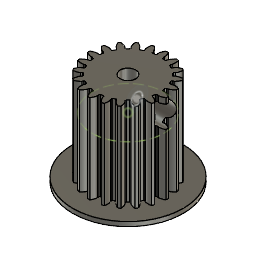
motor gear(pinion) (Autodesk Fusion 360 design; units mm, degrees)
part number: 2025-11-26-00-49-04-497
description: Spur Gear; Module: 1.617; Num Teeth: 20; Pressure Angle: 20.0; Backlash: 0.00 mm
part number: 2025-11-26-00-52-36-103
Autodesk Fusion 360 part; units mm, degrees
(part 1 of 7)
sketch "Sketch1" plane through (0, 0, 0) normal (0, 0, 1) x (1, 0, 0) in component "Spur Gear (20 teeth)"
  circle A0 centre (0, 0) radius 14.1788
  circle A1 centre (0, 0) radius 3.5
extrude "Extrude1" add sketch "Sketch1" along normal blind 15 in component "Spur Gear (20 teeth)"
sketch "Sketch2" plane through (0, 0, 0) normal (0, 0, 1) x (1, 0, 0) in component "Spur Gear (20 teeth)"
  spline S0 degree 5 poles (15.1285, -1.4178) (15.1361, -1.4185) (15.1513, -1.4197) (15.174, -1.4209) (15.2044, -1.4214) (15.2424, -1.4204) (15.2805, -1.4184) (15.3186, -1.4156) (15.3568, -1.4124) (15.395, -1.4089) (15.4332, -1.4052) (15.4714, -1.4011) (15.5096, -1.3966) (15.5478, -1.3915) (15.5861, -1.3859) (15.6243, -1.3797) (15.6625, -1.3731) (15.7008, -1.3662) (15.7391, -1.3589) (15.7773, -1.3513) (15.8155, -1.3434) (15.8538, -1.3352) (15.892, -1.3266) (15.9303, -1.3177) (15.9685, -1.3085) (16.0067, -1.2989) (16.0449, -1.2891) (16.0831, -1.2789) (16.1213, -1.2684) (16.1595, -1.2577) (16.1976, -1.2467) (16.2358, -1.2354) (16.2739, -1.2238) (16.312, -1.2119) (16.3501, -1.1998) (16.3882, -1.1874) (16.4263, -1.1747) (16.4643, -1.1618) (16.5023, -1.1486) (16.5403, -1.1351) (16.5783, -1.1214) (16.6163, -1.1075) (16.6542, -1.0933) (16.6921, -1.0789) (16.73, -1.0642) (16.7678, -1.0493) (16.8057, -1.0341) (16.8435, -1.0187) (16.8813, -1.0031) (16.919, -0.9872) (16.9567, -0.9711) (16.9944, -0.9548) (17.0321, -0.9382) (17.0697, -0.9215) (17.1073, -0.9045) (17.1449, -0.8872) (17.1824, -0.8698) (17.22, -0.8521) (17.2574, -0.8342) (17.2949, -0.8161) (17.3323, -0.7978) (17.3696, -0.7793) (17.407, -0.7606) (17.4443, -0.7416) (17.4815, -0.7225) (17.5187, -0.7031) (17.5559, -0.6835) (17.593, -0.6637) (17.6301, -0.6437) (17.6672, -0.6236) (17.7042, -0.6032) (17.7338, -0.5867) (17.756, -0.5742) (17.7707, -0.5659) (17.7781, -0.5617) knots 0 0 0 0 0 0 0.01428571 0.02857143 0.04285714 0.05714286 0.07142857 0.08571429 0.1 0.11428571 0.12857143 0.14285714 0.15714286 0.17142857 0.18571429 0.2 0.21428571 0.22857143 0.24285714 0.25714286 0.27142857 0.28571429 0.3 0.31428571 0.32857143 0.34285714 0.35714286 0.37142857 0.38571429 0.4 0.41428571 0.42857143 0.44285714 0.45714286 0.47142857 0.48571429 0.5 0.51428571 0.52857143 0.54285714 0.55714286 0.57142857 0.58571429 0.6 0.61428571 0.62857143 0.64285714 0.65714286 0.67142857 0.68571429 0.7 0.71428571 0.72857143 0.74285714 0.75714286 0.77142857 0.78571429 0.8 0.81428571 0.82857143 0.84285714 0.85714286 0.87142857 0.88571429 0.9 0.91428571 0.92857143 0.94285714 0.95714286 0.97142857 0.98571429 1 1 1 1 1 1
  spline S1 degree 5 poles (15.1285, 1.4178) (15.1361, 1.4185) (15.1513, 1.4197) (15.174, 1.4209) (15.2044, 1.4214) (15.2424, 1.4204) (15.2805, 1.4184) (15.3186, 1.4156) (15.3568, 1.4124) (15.395, 1.4089) (15.4332, 1.4052) (15.4714, 1.4011) (15.5096, 1.3966) (15.5478, 1.3915) (15.5861, 1.3859) (15.6243, 1.3797) (15.6625, 1.3731) (15.7008, 1.3662) (15.7391, 1.3589) (15.7773, 1.3513) (15.8155, 1.3434) (15.8538, 1.3352) (15.892, 1.3266) (15.9303, 1.3177) (15.9685, 1.3085) (16.0067, 1.2989) (16.0449, 1.2891) (16.0831, 1.2789) (16.1213, 1.2684) (16.1595, 1.2577) (16.1976, 1.2467) (16.2358, 1.2354) (16.2739, 1.2238) (16.312, 1.2119) (16.3501, 1.1998) (16.3882, 1.1874) (16.4263, 1.1747) (16.4643, 1.1618) (16.5023, 1.1486) (16.5403, 1.1351) (16.5783, 1.1214) (16.6163, 1.1075) (16.6542, 1.0933) (16.6921, 1.0789) (16.73, 1.0642) (16.7678, 1.0493) (16.8057, 1.0341) (16.8435, 1.0187) (16.8813, 1.0031) (16.919, 0.9872) (16.9567, 0.9711) (16.9944, 0.9548) (17.0321, 0.9382) (17.0697, 0.9215) (17.1073, 0.9045) (17.1449, 0.8872) (17.1824, 0.8698) (17.22, 0.8521) (17.2574, 0.8342) (17.2949, 0.8161) (17.3323, 0.7978) (17.3696, 0.7793) (17.407, 0.7606) (17.4443, 0.7416) (17.4815, 0.7225) (17.5187, 0.7031) (17.5559, 0.6835) (17.593, 0.6637) (17.6301, 0.6437) (17.6672, 0.6236) (17.7042, 0.6032) (17.7338, 0.5867) (17.756, 0.5742) (17.7707, 0.5659) (17.7781, 0.5617) knots 0 0 0 0 0 0 0.01428571 0.02857143 0.04285714 0.05714286 0.07142857 0.08571429 0.1 0.11428571 0.12857143 0.14285714 0.15714286 0.17142857 0.18571429 0.2 0.21428571 0.22857143 0.24285714 0.25714286 0.27142857 0.28571429 0.3 0.31428571 0.32857143 0.34285714 0.35714286 0.37142857 0.38571429 0.4 0.41428571 0.42857143 0.44285714 0.45714286 0.47142857 0.48571429 0.5 0.51428571 0.52857143 0.54285714 0.55714286 0.57142857 0.58571429 0.6 0.61428571 0.62857143 0.64285714 0.65714286 0.67142857 0.68571429 0.7 0.71428571 0.72857143 0.74285714 0.75714286 0.77142857 0.78571429 0.8 0.81428571 0.82857143 0.84285714 0.85714286 0.87142857 0.88571429 0.9 0.91428571 0.92857143 0.94285714 0.95714286 0.97142857 0.98571429 1 1 1 1 1 1
  arc A0 (17.7781, -0.5617) -> (17.7781, 0.5617) centre (0, 0) ccw
  line L0 (14.107, -1.323) -> (15.1285, -1.4178)
  line L1 (14.107, 1.323) -> (15.1285, 1.4178)
  line L2 (14.107, -1.323) -> (14.107, 1.323)
  point P0 (15.3147, -1.4158)
  point P1 (15.5023, -1.3974)
  point P2 (15.6908, -1.3679)
  point P3 (15.8799, -1.3293)
  point P4 (16.0695, -1.2825)
  point P5 (16.2594, -1.2281)
  point P6 (16.4496, -1.1667)
  point P7 (16.6398, -1.0986)
  point P8 (16.8301, -1.0241)
  point P9 (17.0203, -0.9434)
  point P10 (17.2102, -0.8567)
  point P11 (17.3999, -0.7641)
  point P12 (17.5893, -0.6657)
  point P13 (15.3147, 1.4158)
  point P14 (15.5023, 1.3974)
  point P15 (15.6908, 1.3679)
  point P16 (15.8799, 1.3293)
  point P17 (16.0695, 1.2825)
  point P18 (16.2594, 1.2281)
  point P19 (16.4496, 1.1667)
  point P20 (16.6398, 1.0986)
  point P21 (16.8301, 1.0241)
  point P22 (17.0203, 0.9434)
  point P23 (17.2102, 0.8567)
  point P24 (17.3999, 0.7641)
  point P25 (17.5893, 0.6657)
extrude "Extrude2" add sketch "Sketch2" along normal blind 15 in component "Spur Gear (20 teeth)"
fillet "Fillet1" radius 0.4 2 edges at (14.1169, -1.3239, 7.5) (14.1169, 1.3239, 7.5) in component "Spur Gear (20 teeth)"
pattern_circular "C-Pattern1" count 20 over 360 about axis through (0, 0, 0) along (0, 0, 1) of "Extrude2", "Fillet1" in component "Spur Gear (20 teeth)"
sketch "Sketch3" plane through (0, 0, 0) normal (0, 0, 1) x (1, 0, 0) in component "Spur Gear (20 teeth)"
  circle A0 centre (0, 0) radius 16.17 construction
sketch "Sketch1 (2)" plane through (0, 0, 0) normal (1, 0, 0) x (0, 1, 0)
  circle A0 through (5, 7.5, 4) (-2.5, 11.8301, 4) (-2.5, 3.1699, 4)
  dimension "d9" = 10
sketch "Sketch2 (2)" plane through (4, 0, 0) normal (1, 0, 0) x (0, 1, 0)
extrude "Extrude7" cut sketch "Sketch1 (2)" along normal blind 16 contours A0 in plane through (4, 0, 0) normal (1, 0, 0) in component "Spur Gear (20 teeth)"
sketch "Sketch4" plane through (4, 0, 0) normal (1, 0, 0) x (0, 1, 0)
  circle A0 centre (0, 7.5) radius 5
  circle A1 centre (0, 7.5) radius 2.5
  dimension "d21" = 5
  constraint concentric A0 A1
  measures "d21" diameter of A1
extrude "Extrude8" cut sketch "Sketch4" against normal blind 16 contours A1 in component "Spur Gear (20 teeth)"
extrude "Extrude10" add 1 faces at (10.5636, 0, 0) along direction (0, 0, -1) blind 10 in component "Spur Gear (20 teeth)"
sketch "Sketch7" plane through (0, 0, -10) normal (0, 0, -1) x (1, 0, 0)
  circle A0 centre (0, 0) radius 3.5
  arc A1 (12.5379, 7.4278) -> (12.3925, 6.8895) centre (12.7421, 7.0839) ccw
  line L0 (12.5379, 7.4278) -> (13.0726, 7.7453)
  spline S0 degree 5 poles (13.0726, 7.7453) (13.0791, 7.7492) (13.0921, 7.7571) (13.1112, 7.7695) (13.1361, 7.787) (13.1663, 7.8101) (13.1959, 7.8342) (13.2251, 7.8589) (13.2541, 7.8839) (13.2829, 7.9091) (13.3116, 7.9346) (13.3402, 7.9603) (13.3684, 7.9864) (13.3963, 8.013) (13.424, 8.0401) (13.4513, 8.0675) (13.4784, 8.0953) (13.5052, 8.1235) (13.5319, 8.1518) (13.5584, 8.1805) (13.5847, 8.2093) (13.6108, 8.2384) (13.6367, 8.2678) (13.6624, 8.2975) (13.6879, 8.3274) (13.7132, 8.3576) (13.7383, 8.3881) (13.7632, 8.4188) (13.788, 8.4497) (13.8125, 8.4808) (13.8369, 8.5122) (13.8611, 8.5437) (13.8852, 8.5755) (13.909, 8.6075) (13.9327, 8.6397) (13.9562, 8.6721) (13.9796, 8.7048) (14.0028, 8.7376) (14.0258, 8.7706) (14.0486, 8.8038) (14.0713, 8.8372) (14.0938, 8.8708) (14.1162, 8.9046) (14.1383, 8.9386) (14.1604, 8.9727) (14.1822, 9.007) (14.2039, 9.0415) (14.2254, 9.0762) (14.2468, 9.1111) (14.268, 9.1461) (14.2891, 9.1813) (14.31, 9.2166) (14.3307, 9.2522) (14.3513, 9.2879) (14.3718, 9.3237) (14.392, 9.3597) (14.4121, 9.3959) (14.4321, 9.4323) (14.4519, 9.4687) (14.4716, 9.5054) (14.491, 9.5422) (14.5104, 9.5791) (14.5296, 9.6162) (14.5486, 9.6535) (14.5675, 9.6909) (14.5862, 9.7284) (14.6048, 9.7661) (14.6232, 9.804) (14.6415, 9.8419) (14.6596, 9.8801) (14.6775, 9.9183) (14.6918, 9.949) (14.7024, 9.9721) (14.7095, 9.9876) (14.713, 9.9953) knots 0 0 0 0 0 0 0.01428571 0.02857143 0.04285714 0.05714286 0.07142857 0.08571429 0.1 0.11428571 0.12857143 0.14285714 0.15714286 0.17142857 0.18571429 0.2 0.21428571 0.22857143 0.24285714 0.25714286 0.27142857 0.28571429 0.3 0.31428571 0.32857143 0.34285714 0.35714286 0.37142857 0.38571429 0.4 0.41428571 0.42857143 0.44285714 0.45714286 0.47142857 0.48571429 0.5 0.51428571 0.52857143 0.54285714 0.55714286 0.57142857 0.58571429 0.6 0.61428571 0.62857143 0.64285714 0.65714286 0.67142857 0.68571429 0.7 0.71428571 0.72857143 0.74285714 0.75714286 0.77142857 0.78571429 0.8 0.81428571 0.82857143 0.84285714 0.85714286 0.87142857 0.88571429 0.9 0.91428571 0.92857143 0.94285714 0.95714286 0.97142857 0.98571429 1 1 1 1 1 1
  arc A2 (14.713, 9.9953) -> (14.0526, 10.9042) centre (0, 0) ccw
  spline S1 degree 5 poles (14.0526, 10.9042) (14.0442, 10.9032) (14.0274, 10.9013) (14.0021, 10.8983) (13.9685, 10.8942) (13.9266, 10.889) (13.8847, 10.8835) (13.8429, 10.8779) (13.8013, 10.8721) (13.7597, 10.8661) (13.7182, 10.8598) (13.6768, 10.8535) (13.6355, 10.8469) (13.5943, 10.8401) (13.5531, 10.8331) (13.5121, 10.8259) (13.4712, 10.8186) (13.4304, 10.811) (13.3896, 10.8033) (13.349, 10.7953) (13.3085, 10.7872) (13.2681, 10.7788) (13.2278, 10.7703) (13.1876, 10.7615) (13.1475, 10.7526) (13.1075, 10.7434) (13.0676, 10.7341) (13.0279, 10.7245) (12.9883, 10.7147) (12.9487, 10.7048) (12.9093, 10.6946) (12.8701, 10.6842) (12.8309, 10.6736) (12.7919, 10.6628) (12.753, 10.6517) (12.7142, 10.6405) (12.6755, 10.629) (12.637, 10.6174) (12.5987, 10.6055) (12.5604, 10.5933) (12.5223, 10.581) (12.4844, 10.5684) (12.4466, 10.5556) (12.4089, 10.5426) (12.3714, 10.5293) (12.334, 10.5158) (12.2968, 10.502) (12.2598, 10.4881) (12.2229, 10.4738) (12.1862, 10.4594) (12.1497, 10.4446) (12.1133, 10.4296) (12.0772, 10.4144) (12.0412, 10.3988) (12.0054, 10.383) (11.9698, 10.3669) (11.9344, 10.3505) (11.8992, 10.3339) (11.8642, 10.3171) (11.8294, 10.2999) (11.7948, 10.2824) (11.7605, 10.2645) (11.7266, 10.2462) (11.693, 10.2274) (11.6597, 10.2082) (11.6266, 10.1888) (11.5937, 10.1691) (11.561, 10.1493) (11.5285, 10.1291) (11.4965, 10.1084) (11.4651, 10.0869) (11.4408, 10.0686) (11.4231, 10.0543) (11.4116, 10.0444) (11.4059, 10.0394) knots -1 -1 -1 -1 -1 -1 -0.98571429 -0.97142857 -0.95714286 -0.94285714 -0.92857143 -0.91428571 -0.9 -0.88571429 -0.87142857 -0.85714286 -0.84285714 -0.82857143 -0.81428571 -0.8 -0.78571429 -0.77142857 -0.75714286 -0.74285714 -0.72857143 -0.71428571 -0.7 -0.68571429 -0.67142857 -0.65714286 -0.64285714 -0.62857143 -0.61428571 -0.6 -0.58571429 -0.57142857 -0.55714286 -0.54285714 -0.52857143 -0.51428571 -0.5 -0.48571429 -0.47142857 -0.45714286 -0.44285714 -0.42857143 -0.41428571 -0.4 -0.38571429 -0.37142857 -0.35714286 -0.34285714 -0.32857143 -0.31428571 -0.3 -0.28571429 -0.27142857 -0.25714286 -0.24285714 -0.22857143 -0.21428571 -0.2 -0.18571429 -0.17142857 -0.15714286 -0.14285714 -0.12857143 -0.11428571 -0.1 -0.08571429 -0.07142857 -0.05714286 -0.04285714 -0.02857143 -0.01428571 0 0 0 0 0 0
  line L1 (11.4059, 10.0394) -> (10.9387, 9.6289)
  arc A3 (10.3818, 9.657) -> (10.9387, 9.6289) centre (10.6747, 9.9294) ccw
  arc A4 (10.3818, 9.657) -> (9.657, 10.3818) centre (0, 0) ccw
  arc A5 (9.6289, 10.9387) -> (9.657, 10.3818) centre (9.9294, 10.6747) ccw
  line L2 (9.6289, 10.9387) -> (10.0394, 11.4059)
  spline S2 degree 5 poles (10.0394, 11.4059) (10.0444, 11.4116) (10.0543, 11.4231) (10.0686, 11.4408) (10.0869, 11.4651) (10.1084, 11.4965) (10.1291, 11.5285) (10.1493, 11.561) (10.1691, 11.5937) (10.1888, 11.6266) (10.2082, 11.6597) (10.2274, 11.693) (10.2462, 11.7266) (10.2645, 11.7605) (10.2824, 11.7948) (10.2999, 11.8294) (10.3171, 11.8642) (10.3339, 11.8992) (10.3505, 11.9344) (10.3669, 11.9698) (10.383, 12.0054) (10.3988, 12.0412) (10.4144, 12.0772) (10.4296, 12.1133) (10.4446, 12.1497) (10.4594, 12.1862) (10.4738, 12.2229) (10.4881, 12.2598) (10.502, 12.2968) (10.5158, 12.334) (10.5293, 12.3714) (10.5426, 12.4089) (10.5556, 12.4466) (10.5684, 12.4844) (10.581, 12.5223) (10.5933, 12.5604) (10.6055, 12.5987) (10.6174, 12.637) (10.629, 12.6755) (10.6405, 12.7142) (10.6517, 12.753) (10.6628, 12.7919) (10.6736, 12.8309) (10.6842, 12.8701) (10.6946, 12.9093) (10.7048, 12.9487) (10.7147, 12.9883) (10.7245, 13.0279) (10.7341, 13.0676) (10.7434, 13.1075) (10.7526, 13.1475) (10.7615, 13.1876) (10.7703, 13.2278) (10.7788, 13.2681) (10.7872, 13.3085) (10.7953, 13.349) (10.8033, 13.3896) (10.811, 13.4304) (10.8186, 13.4712) (10.8259, 13.5121) (10.8331, 13.5531) (10.8401, 13.5943) (10.8469, 13.6355) (10.8535, 13.6768) (10.8598, 13.7182) (10.8661, 13.7597) (10.8721, 13.8013) (10.8779, 13.8429) (10.8835, 13.8847) (10.889, 13.9266) (10.8942, 13.9685) (10.8983, 14.0021) (10.9013, 14.0274) (10.9032, 14.0442) (10.9042, 14.0526) knots 0 0 0 0 0 0 0.01428571 0.02857143 0.04285714 0.05714286 0.07142857 0.08571429 0.1 0.11428571 0.12857143 0.14285714 0.15714286 0.17142857 0.18571429 0.2 0.21428571 0.22857143 0.24285714 0.25714286 0.27142857 0.28571429 0.3 0.31428571 0.32857143 0.34285714 0.35714286 0.37142857 0.38571429 0.4 0.41428571 0.42857143 0.44285714 0.45714286 0.47142857 0.48571429 0.5 0.51428571 0.52857143 0.54285714 0.55714286 0.57142857 0.58571429 0.6 0.61428571 0.62857143 0.64285714 0.65714286 0.67142857 0.68571429 0.7 0.71428571 0.72857143 0.74285714 0.75714286 0.77142857 0.78571429 0.8 0.81428571 0.82857143 0.84285714 0.85714286 0.87142857 0.88571429 0.9 0.91428571 0.92857143 0.94285714 0.95714286 0.97142857 0.98571429 1 1 1 1 1 1
  arc A6 (10.9042, 14.0526) -> (9.9953, 14.713) centre (0, 0) ccw
  spline S3 degree 5 poles (9.9953, 14.713) (9.9876, 14.7095) (9.9721, 14.7024) (9.949, 14.6918) (9.9183, 14.6775) (9.8801, 14.6596) (9.8419, 14.6415) (9.804, 14.6232) (9.7661, 14.6048) (9.7284, 14.5862) (9.6909, 14.5675) (9.6535, 14.5486) (9.6162, 14.5296) (9.5791, 14.5104) (9.5422, 14.491) (9.5054, 14.4716) (9.4687, 14.4519) (9.4323, 14.4321) (9.3959, 14.4121) (9.3597, 14.392) (9.3237, 14.3718) (9.2879, 14.3513) (9.2522, 14.3307) (9.2166, 14.31) (9.1813, 14.2891) (9.1461, 14.268) (9.1111, 14.2468) (9.0762, 14.2254) (9.0415, 14.2039) (9.007, 14.1822) (8.9727, 14.1604) (8.9386, 14.1383) (8.9046, 14.1162) (8.8708, 14.0938) (8.8372, 14.0713) (8.8038, 14.0486) (8.7706, 14.0258) (8.7376, 14.0028) (8.7048, 13.9796) (8.6721, 13.9562) (8.6397, 13.9327) (8.6075, 13.909) (8.5755, 13.8852) (8.5437, 13.8611) (8.5122, 13.8369) (8.4808, 13.8125) (8.4497, 13.788) (8.4188, 13.7632) (8.3881, 13.7383) (8.3576, 13.7132) (8.3274, 13.6879) (8.2975, 13.6624) (8.2678, 13.6367) (8.2384, 13.6108) (8.2093, 13.5847) (8.1805, 13.5584) (8.1518, 13.5319) (8.1235, 13.5052) (8.0953, 13.4784) (8.0675, 13.4513) (8.0401, 13.424) (8.013, 13.3963) (7.9864, 13.3684) (7.9603, 13.3402) (7.9346, 13.3116) (7.9091, 13.2829) (7.8839, 13.2541) (7.8589, 13.2251) (7.8342, 13.1959) (7.8101, 13.1663) (7.787, 13.1361) (7.7695, 13.1112) (7.7571, 13.0921) (7.7492, 13.0791) (7.7453, 13.0726) knots -1 -1 -1 -1 -1 -1 -0.98571429 -0.97142857 -0.95714286 -0.94285714 -0.92857143 -0.91428571 -0.9 -0.88571429 -0.87142857 -0.85714286 -0.84285714 -0.82857143 -0.81428571 -0.8 -0.78571429 -0.77142857 -0.75714286 -0.74285714 -0.72857143 -0.71428571 -0.7 -0.68571429 -0.67142857 -0.65714286 -0.64285714 -0.62857143 -0.61428571 -0.6 -0.58571429 -0.57142857 -0.55714286 -0.54285714 -0.52857143 -0.51428571 -0.5 -0.48571429 -0.47142857 -0.45714286 -0.44285714 -0.42857143 -0.41428571 -0.4 -0.38571429 -0.37142857 -0.35714286 -0.34285714 -0.32857143 -0.31428571 -0.3 -0.28571429 -0.27142857 -0.25714286 -0.24285714 -0.22857143 -0.21428571 -0.2 -0.18571429 -0.17142857 -0.15714286 -0.14285714 -0.12857143 -0.11428571 -0.1 -0.08571429 -0.07142857 -0.05714286 -0.04285714 -0.02857143 -0.01428571 0 0 0 0 0 0
  line L3 (7.7453, 13.0726) -> (7.4278, 12.5379)
  arc A7 (6.8895, 12.3925) -> (7.4278, 12.5379) centre (7.0839, 12.7421) ccw
  arc A8 (6.8895, 12.3925) -> (5.9762, 12.8578) centre (0, 0) ccw
  arc A9 (5.7774, 13.3788) -> (5.9762, 12.8578) centre (6.1448, 13.2206) ccw
  line L4 (5.7774, 13.3788) -> (6.0234, 13.95)
  spline S4 degree 5 poles (6.0234, 13.95) (6.0264, 13.957) (6.0322, 13.971) (6.0404, 13.9923) (6.0502, 14.021) (6.0611, 14.0575) (6.0709, 14.0943) (6.08, 14.1315) (6.0888, 14.1687) (6.0973, 14.2061) (6.1055, 14.2436) (6.1135, 14.2812) (6.121, 14.3189) (6.1279, 14.3569) (6.1344, 14.395) (6.1404, 14.4332) (6.1459, 14.4717) (6.1511, 14.5102) (6.156, 14.5488) (6.1606, 14.5875) (6.1649, 14.6264) (6.1689, 14.6653) (6.1726, 14.7043) (6.176, 14.7434) (6.179, 14.7826) (6.1817, 14.8219) (6.1841, 14.8613) (6.1862, 14.9008) (6.1881, 14.9403) (6.1897, 14.9799) (6.191, 15.0196) (6.192, 15.0594) (6.1928, 15.0992) (6.1933, 15.1392) (6.1935, 15.1791) (6.1935, 15.2192) (6.1932, 15.2593) (6.1927, 15.2995) (6.1919, 15.3397) (6.1908, 15.38) (6.1895, 15.4204) (6.188, 15.4608) (6.1862, 15.5012) (6.1842, 15.5417) (6.182, 15.5823) (6.1795, 15.6229) (6.1767, 15.6636) (6.1738, 15.7043) (6.1706, 15.7451) (6.1672, 15.7859) (6.1635, 15.8267) (6.1596, 15.8676) (6.1555, 15.9086) (6.1512, 15.9495) (6.1466, 15.9906) (6.1419, 16.0316) (6.1369, 16.0727) (6.1317, 16.1138) (6.1262, 16.155) (6.1206, 16.1962) (6.1147, 16.2374) (6.1087, 16.2787) (6.1024, 16.32) (6.0959, 16.3613) (6.0892, 16.4027) (6.0823, 16.444) (6.0751, 16.4854) (6.0678, 16.5269) (6.0602, 16.5683) (6.0525, 16.6098) (6.0445, 16.6513) (6.038, 16.6846) (6.033, 16.7095) (6.0297, 16.7261) (6.028, 16.7344) knots 0 0 0 0 0 0 0.01428571 0.02857143 0.04285714 0.05714286 0.07142857 0.08571429 0.1 0.11428571 0.12857143 0.14285714 0.15714286 0.17142857 0.18571429 0.2 0.21428571 0.22857143 0.24285714 0.25714286 0.27142857 0.28571429 0.3 0.31428571 0.32857143 0.34285714 0.35714286 0.37142857 0.38571429 0.4 0.41428571 0.42857143 0.44285714 0.45714286 0.47142857 0.48571429 0.5 0.51428571 0.52857143 0.54285714 0.55714286 0.57142857 0.58571429 0.6 0.61428571 0.62857143 0.64285714 0.65714286 0.67142857 0.68571429 0.7 0.71428571 0.72857143 0.74285714 0.75714286 0.77142857 0.78571429 0.8 0.81428571 0.82857143 0.84285714 0.85714286 0.87142857 0.88571429 0.9 0.91428571 0.92857143 0.94285714 0.95714286 0.97142857 0.98571429 1 1 1 1 1 1
  arc A10 (6.028, 16.7344) -> (4.9595, 17.0816) centre (0, 0) ccw
  spline S5 degree 5 poles (4.9595, 17.0816) (4.9533, 17.0759) (4.9408, 17.0644) (4.9221, 17.0471) (4.8973, 17.0241) (4.8664, 16.9952) (4.8358, 16.9662) (4.8053, 16.9371) (4.775, 16.9079) (4.7449, 16.8786) (4.715, 16.8492) (4.6853, 16.8196) (4.6557, 16.79) (4.6263, 16.7603) (4.5972, 16.7305) (4.5682, 16.7006) (4.5394, 16.6706) (4.5108, 16.6405) (4.4825, 16.6103) (4.4543, 16.5799) (4.4263, 16.5495) (4.3985, 16.519) (4.3709, 16.4884) (4.3435, 16.4577) (4.3163, 16.4269) (4.2894, 16.396) (4.2626, 16.365) (4.2361, 16.3339) (4.2098, 16.3027) (4.1836, 16.2714) (4.1577, 16.24) (4.1321, 16.2085) (4.1066, 16.1769) (4.0814, 16.1452) (4.0564, 16.1134) (4.0317, 16.0816) (4.0071, 16.0496) (3.9828, 16.0175) (3.9588, 15.9853) (3.935, 15.953) (3.9114, 15.9206) (3.8881, 15.8882) (3.865, 15.8556) (3.8422, 15.8229) (3.8197, 15.7901) (3.7974, 15.7572) (3.7754, 15.7242) (3.7537, 15.6911) (3.7322, 15.658) (3.711, 15.6247) (3.6901, 15.5913) (3.6695, 15.5578) (3.6492, 15.5242) (3.6293, 15.4904) (3.6096, 15.4566) (3.5903, 15.4227) (3.5713, 15.3886) (3.5525, 15.3545) (3.5341, 15.3203) (3.516, 15.2859) (3.4983, 15.2515) (3.4811, 15.2168) (3.4645, 15.1821) (3.4484, 15.1471) (3.4327, 15.112) (3.4173, 15.0769) (3.4023, 15.0416) (3.3874, 15.0063) (3.373, 14.9709) (3.3592, 14.9353) (3.3466, 14.8995) (3.3376, 14.8704) (3.3318, 14.8484) (3.3282, 14.8336) (3.3266, 14.8262) knots -1 -1 -1 -1 -1 -1 -0.98571429 -0.97142857 -0.95714286 -0.94285714 -0.92857143 -0.91428571 -0.9 -0.88571429 -0.87142857 -0.85714286 -0.84285714 -0.82857143 -0.81428571 -0.8 -0.78571429 -0.77142857 -0.75714286 -0.74285714 -0.72857143 -0.71428571 -0.7 -0.68571429 -0.67142857 -0.65714286 -0.64285714 -0.62857143 -0.61428571 -0.6 -0.58571429 -0.57142857 -0.55714286 -0.54285714 -0.52857143 -0.51428571 -0.5 -0.48571429 -0.47142857 -0.45714286 -0.44285714 -0.42857143 -0.41428571 -0.4 -0.38571429 -0.37142857 -0.35714286 -0.34285714 -0.32857143 -0.31428571 -0.3 -0.28571429 -0.27142857 -0.25714286 -0.24285714 -0.22857143 -0.21428571 -0.2 -0.18571429 -0.17142857 -0.15714286 -0.14285714 -0.12857143 -0.11428571 -0.1 -0.08571429 -0.07142857 -0.05714286 -0.04285714 -0.02857143 -0.01428571 0 0 0 0 0 0
  line L5 (3.3266, 14.8262) -> (3.1899, 14.2195)
  arc A11 (2.7228, 13.9149) -> (3.1899, 14.2195) centre (2.7996, 14.3075) ccw
  arc A12 (2.7228, 13.9149) -> (1.7104, 14.0753) centre (0, 0) ccw
  arc A13 (1.3603, 14.5093) -> (1.7104, 14.0753) centre (1.7586, 14.4723) ccw
  line L6 (1.3603, 14.5093) -> (1.4178, 15.1285)
  spline S6 degree 5 poles (1.4178, 15.1285) (1.4185, 15.1361) (1.4197, 15.1513) (1.4209, 15.174) (1.4214, 15.2044) (1.4204, 15.2424) (1.4184, 15.2805) (1.4156, 15.3186) (1.4124, 15.3568) (1.4089, 15.395) (1.4052, 15.4332) (1.4011, 15.4714) (1.3966, 15.5096) (1.3915, 15.5478) (1.3859, 15.5861) (1.3797, 15.6243) (1.3731, 15.6625) (1.3662, 15.7008) (1.3589, 15.7391) (1.3513, 15.7773) (1.3434, 15.8155) (1.3352, 15.8538) (1.3266, 15.892) (1.3177, 15.9303) (1.3085, 15.9685) (1.2989, 16.0067) (1.2891, 16.0449) (1.2789, 16.0831) (1.2684, 16.1213) (1.2577, 16.1595) (1.2467, 16.1976) (1.2354, 16.2358) (1.2238, 16.2739) (1.2119, 16.312) (1.1998, 16.3501) (1.1874, 16.3882) (1.1747, 16.4263) (1.1618, 16.4643) (1.1486, 16.5023) (1.1351, 16.5403) (1.1214, 16.5783) (1.1075, 16.6163) (1.0933, 16.6542) (1.0789, 16.6921) (1.0642, 16.73) (1.0493, 16.7678) (1.0341, 16.8057) (1.0187, 16.8435) (1.0031, 16.8813) (0.9872, 16.919) (0.9711, 16.9567) (0.9548, 16.9944) (0.9382, 17.0321) (0.9215, 17.0697) (0.9045, 17.1073) (0.8872, 17.1449) (0.8698, 17.1824) (0.8521, 17.22) (0.8342, 17.2574) (0.8161, 17.2949) (0.7978, 17.3323) (0.7793, 17.3696) (0.7606, 17.407) (0.7416, 17.4443) (0.7225, 17.4815) (0.7031, 17.5187) (0.6835, 17.5559) (0.6637, 17.593) (0.6437, 17.6301) (0.6236, 17.6672) (0.6032, 17.7042) (0.5867, 17.7338) (0.5742, 17.756) (0.5659, 17.7707) (0.5617, 17.7781) knots 0 0 0 0 0 0 0.01428571 0.02857143 0.04285714 0.05714286 0.07142857 0.08571429 0.1 0.11428571 0.12857143 0.14285714 0.15714286 0.17142857 0.18571429 0.2 0.21428571 0.22857143 0.24285714 0.25714286 0.27142857 0.28571429 0.3 0.31428571 0.32857143 0.34285714 0.35714286 0.37142857 0.38571429 0.4 0.41428571 0.42857143 0.44285714 0.45714286 0.47142857 0.48571429 0.5 0.51428571 0.52857143 0.54285714 0.55714286 0.57142857 0.58571429 0.6 0.61428571 0.62857143 0.64285714 0.65714286 0.67142857 0.68571429 0.7 0.71428571 0.72857143 0.74285714 0.75714286 0.77142857 0.78571429 0.8 0.81428571 0.82857143 0.84285714 0.85714286 0.87142857 0.88571429 0.9 0.91428571 0.92857143 0.94285714 0.95714286 0.97142857 0.98571429 1 1 1 1 1 1
  arc A14 (0.5617, 17.7781) -> (-0.5617, 17.7781) centre (0, 0) ccw
  spline S7 degree 5 poles (-0.5617, 17.7781) (-0.5659, 17.7707) (-0.5742, 17.756) (-0.5867, 17.7338) (-0.6032, 17.7042) (-0.6236, 17.6672) (-0.6437, 17.6301) (-0.6637, 17.593) (-0.6835, 17.5559) (-0.7031, 17.5187) (-0.7225, 17.4815) (-0.7416, 17.4443) (-0.7606, 17.407) (-0.7793, 17.3696) (-0.7978, 17.3323) (-0.8161, 17.2949) (-0.8342, 17.2574) (-0.8521, 17.22) (-0.8698, 17.1824) (-0.8872, 17.1449) (-0.9045, 17.1073) (-0.9215, 17.0697) (-0.9382, 17.0321) (-0.9548, 16.9944) (-0.9711, 16.9567) (-0.9872, 16.919) (-1.0031, 16.8813) (-1.0187, 16.8435) (-1.0341, 16.8057) (-1.0493, 16.7678) (-1.0642, 16.73) (-1.0789, 16.6921) (-1.0933, 16.6542) (-1.1075, 16.6163) (-1.1214, 16.5783) (-1.1351, 16.5403) (-1.1486, 16.5023) (-1.1618, 16.4643) (-1.1747, 16.4263) (-1.1874, 16.3882) (-1.1998, 16.3501) (-1.2119, 16.312) (-1.2238, 16.2739) (-1.2354, 16.2358) (-1.2467, 16.1976) (-1.2577, 16.1595) (-1.2684, 16.1213) (-1.2789, 16.0831) (-1.2891, 16.0449) (-1.2989, 16.0067) (-1.3085, 15.9685) (-1.3177, 15.9303) (-1.3266, 15.892) (-1.3352, 15.8538) (-1.3434, 15.8155) (-1.3513, 15.7773) (-1.3589, 15.7391) (-1.3662, 15.7008) (-1.3731, 15.6625) (-1.3797, 15.6243) (-1.3859, 15.5861) (-1.3915, 15.5478) (-1.3966, 15.5096) (-1.4011, 15.4714) (-1.4052, 15.4332) (-1.4089, 15.395) (-1.4124, 15.3568) (-1.4156, 15.3186) (-1.4184, 15.2805) (-1.4204, 15.2424) (-1.4214, 15.2044) (-1.4209, 15.174) (-1.4197, 15.1513) (-1.4185, 15.1361) (-1.4178, 15.1285) knots -1 -1 -1 -1 -1 -1 -0.98571429 -0.97142857 -0.95714286 -0.94285714 -0.92857143 -0.91428571 -0.9 -0.88571429 -0.87142857 -0.85714286 -0.84285714 -0.82857143 -0.81428571 -0.8 -0.78571429 -0.77142857 -0.75714286 -0.74285714 -0.72857143 -0.71428571 -0.7 -0.68571429 -0.67142857 -0.65714286 -0.64285714 -0.62857143 -0.61428571 -0.6 -0.58571429 -0.57142857 -0.55714286 -0.54285714 -0.52857143 -0.51428571 -0.5 -0.48571429 -0.47142857 -0.45714286 -0.44285714 -0.42857143 -0.41428571 -0.4 -0.38571429 -0.37142857 -0.35714286 -0.34285714 -0.32857143 -0.31428571 -0.3 -0.28571429 -0.27142857 -0.25714286 -0.24285714 -0.22857143 -0.21428571 -0.2 -0.18571429 -0.17142857 -0.15714286 -0.14285714 -0.12857143 -0.11428571 -0.1 -0.08571429 -0.07142857 -0.05714286 -0.04285714 -0.02857143 -0.01428571 0 0 0 0 0 0
  line L7 (-1.4178, 15.1285) -> (-1.3603, 14.5093)
  arc A15 (-1.7104, 14.0753) -> (-1.3603, 14.5093) centre (-1.7586, 14.4723) ccw
  arc A16 (-1.7104, 14.0753) -> (-2.7228, 13.9149) centre (0, 0) ccw
  arc A17 (-3.1899, 14.2195) -> (-2.7228, 13.9149) centre (-2.7996, 14.3075) ccw
  line L8 (-3.1899, 14.2195) -> (-3.3266, 14.8262)
  spline S8 degree 5 poles (-3.3266, 14.8262) (-3.3282, 14.8336) (-3.3318, 14.8484) (-3.3376, 14.8704) (-3.3466, 14.8995) (-3.3592, 14.9353) (-3.373, 14.9709) (-3.3874, 15.0063) (-3.4023, 15.0416) (-3.4173, 15.0769) (-3.4327, 15.112) (-3.4484, 15.1471) (-3.4645, 15.1821) (-3.4811, 15.2168) (-3.4983, 15.2515) (-3.516, 15.2859) (-3.5341, 15.3203) (-3.5525, 15.3545) (-3.5713, 15.3886) (-3.5903, 15.4227) (-3.6096, 15.4566) (-3.6293, 15.4904) (-3.6492, 15.5242) (-3.6695, 15.5578) (-3.6901, 15.5913) (-3.711, 15.6247) (-3.7322, 15.658) (-3.7537, 15.6911) (-3.7754, 15.7242) (-3.7974, 15.7572) (-3.8197, 15.7901) (-3.8422, 15.8229) (-3.865, 15.8556) (-3.8881, 15.8882) (-3.9114, 15.9206) (-3.935, 15.953) (-3.9588, 15.9853) (-3.9828, 16.0175) (-4.0071, 16.0496) (-4.0317, 16.0816) (-4.0564, 16.1134) (-4.0814, 16.1452) (-4.1066, 16.1769) (-4.1321, 16.2085) (-4.1577, 16.24) (-4.1836, 16.2714) (-4.2098, 16.3027) (-4.2361, 16.3339) (-4.2626, 16.365) (-4.2894, 16.396) (-4.3163, 16.4269) (-4.3435, 16.4577) (-4.3709, 16.4884) (-4.3985, 16.519) (-4.4263, 16.5495) (-4.4543, 16.5799) (-4.4825, 16.6103) (-4.5108, 16.6405) (-4.5394, 16.6706) (-4.5682, 16.7006) (-4.5972, 16.7305) (-4.6263, 16.7603) (-4.6557, 16.79) (-4.6853, 16.8196) (-4.715, 16.8492) (-4.7449, 16.8786) (-4.775, 16.9079) (-4.8053, 16.9371) (-4.8358, 16.9662) (-4.8664, 16.9952) (-4.8973, 17.0241) (-4.9221, 17.0471) (-4.9408, 17.0644) (-4.9533, 17.0759) (-4.9595, 17.0816) knots 0 0 0 0 0 0 0.01428571 0.02857143 0.04285714 0.05714286 0.07142857 0.08571429 0.1 0.11428571 0.12857143 0.14285714 0.15714286 0.17142857 0.18571429 0.2 0.21428571 0.22857143 0.24285714 0.25714286 0.27142857 0.28571429 0.3 0.31428571 0.32857143 0.34285714 0.35714286 0.37142857 0.38571429 0.4 0.41428571 0.42857143 0.44285714 0.45714286 0.47142857 0.48571429 0.5 0.51428571 0.52857143 0.54285714 0.55714286 0.57142857 0.58571429 0.6 0.61428571 0.62857143 0.64285714 0.65714286 0.67142857 0.68571429 0.7 0.71428571 0.72857143 0.74285714 0.75714286 0.77142857 0.78571429 0.8 0.81428571 0.82857143 0.84285714 0.85714286 0.87142857 0.88571429 0.9 0.91428571 0.92857143 0.94285714 0.95714286 0.97142857 0.98571429 1 1 1 1 1 1
  arc A18 (-4.9595, 17.0816) -> (-6.028, 16.7344) centre (0, 0) ccw
  spline S9 degree 5 poles (-6.028, 16.7344) (-6.0297, 16.7261) (-6.033, 16.7095) (-6.038, 16.6846) (-6.0445, 16.6513) (-6.0525, 16.6098) (-6.0602, 16.5683) (-6.0678, 16.5269) (-6.0751, 16.4854) (-6.0823, 16.444) (-6.0892, 16.4027) (-6.0959, 16.3613) (-6.1024, 16.32) (-6.1087, 16.2787) (-6.1147, 16.2374) (-6.1206, 16.1962) (-6.1262, 16.155) (-6.1317, 16.1138) (-6.1369, 16.0727) (-6.1419, 16.0316) (-6.1466, 15.9906) (-6.1512, 15.9495) (-6.1555, 15.9086) (-6.1596, 15.8676) (-6.1635, 15.8267) (-6.1672, 15.7859) (-6.1706, 15.7451) (-6.1738, 15.7043) (-6.1767, 15.6636) (-6.1795, 15.6229) (-6.182, 15.5823) (-6.1842, 15.5417) (-6.1862, 15.5012) (-6.188, 15.4608) (-6.1895, 15.4204) (-6.1908, 15.38) (-6.1919, 15.3397) (-6.1927, 15.2995) (-6.1932, 15.2593) (-6.1935, 15.2192) (-6.1935, 15.1791) (-6.1933, 15.1392) (-6.1928, 15.0992) (-6.192, 15.0594) (-6.191, 15.0196) (-6.1897, 14.9799) (-6.1881, 14.9403) (-6.1862, 14.9008) (-6.1841, 14.8613) (-6.1817, 14.8219) (-6.179, 14.7826) (-6.176, 14.7434) (-6.1726, 14.7043) (-6.1689, 14.6653) (-6.1649, 14.6264) (-6.1606, 14.5875) (-6.156, 14.5488) (-6.1511, 14.5102) (-6.1459, 14.4717) (-6.1404, 14.4332) (-6.1344, 14.395) (-6.1279, 14.3569) (-6.121, 14.3189) (-6.1135, 14.2812) (-6.1055, 14.2436) (-6.0973, 14.2061) (-6.0888, 14.1687) (-6.08, 14.1315) (-6.0709, 14.0943) (-6.0611, 14.0575) (-6.0502, 14.021) (-6.0404, 13.9923) (-6.0322, 13.971) (-6.0264, 13.957) (-6.0234, 13.95) knots -1 -1 -1 -1 -1 -1 -0.98571429 -0.97142857 -0.95714286 -0.94285714 -0.92857143 -0.91428571 -0.9 -0.88571429 -0.87142857 -0.85714286 -0.84285714 -0.82857143 -0.81428571 -0.8 -0.78571429 -0.77142857 -0.75714286 -0.74285714 -0.72857143 -0.71428571 -0.7 -0.68571429 -0.67142857 -0.65714286 -0.64285714 -0.62857143 -0.61428571 -0.6 -0.58571429 -0.57142857 -0.55714286 -0.54285714 -0.52857143 -0.51428571 -0.5 -0.48571429 -0.47142857 -0.45714286 -0.44285714 -0.42857143 -0.41428571 -0.4 -0.38571429 -0.37142857 -0.35714286 -0.34285714 -0.32857143 -0.31428571 -0.3 -0.28571429 -0.27142857 -0.25714286 -0.24285714 -0.22857143 -0.21428571 -0.2 -0.18571429 -0.17142857 -0.15714286 -0.14285714 -0.12857143 -0.11428571 -0.1 -0.08571429 -0.07142857 -0.05714286 -0.04285714 -0.02857143 -0.01428571 0 0 0 0 0 0
  line L9 (-6.0234, 13.95) -> (-5.7774, 13.3788)
  arc A19 (-5.9762, 12.8578) -> (-5.7774, 13.3788) centre (-6.1448, 13.2206) ccw
  arc A20 (-5.9762, 12.8578) -> (-6.8895, 12.3925) centre (0, 0) ccw
  arc A21 (-7.4278, 12.5379) -> (-6.8895, 12.3925) centre (-7.0839, 12.7421) ccw
  line L10 (-7.4278, 12.5379) -> (-7.7453, 13.0726)
  spline S10 degree 5 poles (-7.7453, 13.0726) (-7.7492, 13.0791) (-7.7571, 13.0921) (-7.7695, 13.1112) (-7.787, 13.1361) (-7.8101, 13.1663) (-7.8342, 13.1959) (-7.8589, 13.2251) (-7.8839, 13.2541) (-7.9091, 13.2829) (-7.9346, 13.3116) (-7.9603, 13.3402) (-7.9864, 13.3684) (-8.013, 13.3963) (-8.0401, 13.424) (-8.0675, 13.4513) (-8.0953, 13.4784) (-8.1235, 13.5052) (-8.1518, 13.5319) (-8.1805, 13.5584) (-8.2093, 13.5847) (-8.2384, 13.6108) (-8.2678, 13.6367) (-8.2975, 13.6624) (-8.3274, 13.6879) (-8.3576, 13.7132) (-8.3881, 13.7383) (-8.4188, 13.7632) (-8.4497, 13.788) (-8.4808, 13.8125) (-8.5122, 13.8369) (-8.5437, 13.8611) (-8.5755, 13.8852) (-8.6075, 13.909) (-8.6397, 13.9327) (-8.6721, 13.9562) (-8.7048, 13.9796) (-8.7376, 14.0028) (-8.7706, 14.0258) (-8.8038, 14.0486) (-8.8372, 14.0713) (-8.8708, 14.0938) (-8.9046, 14.1162) (-8.9386, 14.1383) (-8.9727, 14.1604) (-9.007, 14.1822) (-9.0415, 14.2039) (-9.0762, 14.2254) (-9.1111, 14.2468) (-9.1461, 14.268) (-9.1813, 14.2891) (-9.2166, 14.31) (-9.2522, 14.3307) (-9.2879, 14.3513) (-9.3237, 14.3718) (-9.3597, 14.392) (-9.3959, 14.4121) (-9.4323, 14.4321) (-9.4687, 14.4519) (-9.5054, 14.4716) (-9.5422, 14.491) (-9.5791, 14.5104) (-9.6162, 14.5296) (-9.6535, 14.5486) (-9.6909, 14.5675) (-9.7284, 14.5862) (-9.7661, 14.6048) (-9.804, 14.6232) (-9.8419, 14.6415) (-9.8801, 14.6596) (-9.9183, 14.6775) (-9.949, 14.6918) (-9.9721, 14.7024) (-9.9876, 14.7095) (-9.9953, 14.713) knots 0 0 0 0 0 0 0.01428571 0.02857143 0.04285714 0.05714286 0.07142857 0.08571429 0.1 0.11428571 0.12857143 0.14285714 0.15714286 0.17142857 0.18571429 0.2 0.21428571 0.22857143 0.24285714 0.25714286 0.27142857 0.28571429 0.3 0.31428571 0.32857143 0.34285714 0.35714286 0.37142857 0.38571429 0.4 0.41428571 0.42857143 0.44285714 0.45714286 0.47142857 0.48571429 0.5 0.51428571 0.52857143 0.54285714 0.55714286 0.57142857 0.58571429 0.6 0.61428571 0.62857143 0.64285714 0.65714286 0.67142857 0.68571429 0.7 0.71428571 0.72857143 0.74285714 0.75714286 0.77142857 0.78571429 0.8 0.81428571 0.82857143 0.84285714 0.85714286 0.87142857 0.88571429 0.9 0.91428571 0.92857143 0.94285714 0.95714286 0.97142857 0.98571429 1 1 1 1 1 1
  arc A22 (-9.9953, 14.713) -> (-10.9042, 14.0526) centre (0, 0) ccw
  spline S11 degree 5 poles (-10.9042, 14.0526) (-10.9032, 14.0442) (-10.9013, 14.0274) (-10.8983, 14.0021) (-10.8942, 13.9685) (-10.889, 13.9266) (-10.8835, 13.8847) (-10.8779, 13.8429) (-10.8721, 13.8013) (-10.8661, 13.7597) (-10.8598, 13.7182) (-10.8535, 13.6768) (-10.8469, 13.6355) (-10.8401, 13.5943) (-10.8331, 13.5531) (-10.8259, 13.5121) (-10.8186, 13.4712) (-10.811, 13.4304) (-10.8033, 13.3896) (-10.7953, 13.349) (-10.7872, 13.3085) (-10.7788, 13.2681) (-10.7703, 13.2278) (-10.7615, 13.1876) (-10.7526, 13.1475) (-10.7434, 13.1075) (-10.7341, 13.0676) (-10.7245, 13.0279) (-10.7147, 12.9883) (-10.7048, 12.9487) (-10.6946, 12.9093) (-10.6842, 12.8701) (-10.6736, 12.8309) (-10.6628, 12.7919) (-10.6517, 12.753) (-10.6405, 12.7142) (-10.629, 12.6755) (-10.6174, 12.637) (-10.6055, 12.5987) (-10.5933, 12.5604) (-10.581, 12.5223) (-10.5684, 12.4844) (-10.5556, 12.4466) (-10.5426, 12.4089) (-10.5293, 12.3714) (-10.5158, 12.334) (-10.502, 12.2968) (-10.4881, 12.2598) (-10.4738, 12.2229) (-10.4594, 12.1862) (-10.4446, 12.1497) (-10.4296, 12.1133) (-10.4144, 12.0772) (-10.3988, 12.0412) (-10.383, 12.0054) (-10.3669, 11.9698) (-10.3505, 11.9344) (-10.3339, 11.8992) (-10.3171, 11.8642) (-10.2999, 11.8294) (-10.2824, 11.7948) (-10.2645, 11.7605) (-10.2462, 11.7266) (-10.2274, 11.693) (-10.2082, 11.6597) (-10.1888, 11.6266) (-10.1691, 11.5937) (-10.1493, 11.561) (-10.1291, 11.5285) (-10.1084, 11.4965) (-10.0869, 11.4651) (-10.0686, 11.4408) (-10.0543, 11.4231) (-10.0444, 11.4116) (-10.0394, 11.4059) knots -1 -1 -1 -1 -1 -1 -0.98571429 -0.97142857 -0.95714286 -0.94285714 -0.92857143 -0.91428571 -0.9 -0.88571429 -0.87142857 -0.85714286 -0.84285714 -0.82857143 -0.81428571 -0.8 -0.78571429 -0.77142857 -0.75714286 -0.74285714 -0.72857143 -0.71428571 -0.7 -0.68571429 -0.67142857 -0.65714286 -0.64285714 -0.62857143 -0.61428571 -0.6 -0.58571429 -0.57142857 -0.55714286 -0.54285714 -0.52857143 -0.51428571 -0.5 -0.48571429 -0.47142857 -0.45714286 -0.44285714 -0.42857143 -0.41428571 -0.4 -0.38571429 -0.37142857 -0.35714286 -0.34285714 -0.32857143 -0.31428571 -0.3 -0.28571429 -0.27142857 -0.25714286 -0.24285714 -0.22857143 -0.21428571 -0.2 -0.18571429 -0.17142857 -0.15714286 -0.14285714 -0.12857143 -0.11428571 -0.1 -0.08571429 -0.07142857 -0.05714286 -0.04285714 -0.02857143 -0.01428571 0 0 0 0 0 0
  line L11 (-10.0394, 11.4059) -> (-9.6289, 10.9387)
  arc A23 (-9.657, 10.3818) -> (-9.6289, 10.9387) centre (-9.9294, 10.6747) ccw
  arc A24 (-9.657, 10.3818) -> (-10.3818, 9.657) centre (0, 0) ccw
  arc A25 (-10.9387, 9.6289) -> (-10.3818, 9.657) centre (-10.6747, 9.9294) ccw
  line L12 (-10.9387, 9.6289) -> (-11.4059, 10.0394)
  spline S12 degree 5 poles (-11.4059, 10.0394) (-11.4116, 10.0444) (-11.4231, 10.0543) (-11.4408, 10.0686) (-11.4651, 10.0869) (-11.4965, 10.1084) (-11.5285, 10.1291) (-11.561, 10.1493) (-11.5937, 10.1691) (-11.6266, 10.1888) (-11.6597, 10.2082) (-11.693, 10.2274) (-11.7266, 10.2462) (-11.7605, 10.2645) (-11.7948, 10.2824) (-11.8294, 10.2999) (-11.8642, 10.3171) (-11.8992, 10.3339) (-11.9344, 10.3505) (-11.9698, 10.3669) (-12.0054, 10.383) (-12.0412, 10.3988) (-12.0772, 10.4144) (-12.1133, 10.4296) (-12.1497, 10.4446) (-12.1862, 10.4594) (-12.2229, 10.4738) (-12.2598, 10.4881) (-12.2968, 10.502) (-12.334, 10.5158) (-12.3714, 10.5293) (-12.4089, 10.5426) (-12.4466, 10.5556) (-12.4844, 10.5684) (-12.5223, 10.581) (-12.5604, 10.5933) (-12.5987, 10.6055) (-12.637, 10.6174) (-12.6755, 10.629) (-12.7142, 10.6405) (-12.753, 10.6517) (-12.7919, 10.6628) (-12.8309, 10.6736) (-12.8701, 10.6842) (-12.9093, 10.6946) (-12.9487, 10.7048) (-12.9883, 10.7147) (-13.0279, 10.7245) (-13.0676, 10.7341) (-13.1075, 10.7434) (-13.1475, 10.7526) (-13.1876, 10.7615) (-13.2278, 10.7703) (-13.2681, 10.7788) (-13.3085, 10.7872) (-13.349, 10.7953) (-13.3896, 10.8033) (-13.4304, 10.811) (-13.4712, 10.8186) (-13.5121, 10.8259) (-13.5531, 10.8331) (-13.5943, 10.8401) (-13.6355, 10.8469) (-13.6768, 10.8535) (-13.7182, 10.8598) (-13.7597, 10.8661) (-13.8013, 10.8721) (-13.8429, 10.8779) (-13.8847, 10.8835) (-13.9266, 10.889) (-13.9685, 10.8942) (-14.0021, 10.8983) (-14.0274, 10.9013) (-14.0442, 10.9032) (-14.0526, 10.9042) knots 0 0 0 0 0 0 0.01428571 0.02857143 0.04285714 0.05714286 0.07142857 0.08571429 0.1 0.11428571 0.12857143 0.14285714 0.15714286 0.17142857 0.18571429 0.2 0.21428571 0.22857143 0.24285714 0.25714286 0.27142857 0.28571429 0.3 0.31428571 0.32857143 0.34285714 0.35714286 0.37142857 0.38571429 0.4 0.41428571 0.42857143 0.44285714 0.45714286 0.47142857 0.48571429 0.5 0.51428571 0.52857143 0.54285714 0.55714286 0.57142857 0.58571429 0.6 0.61428571 0.62857143 0.64285714 0.65714286 0.67142857 0.68571429 0.7 0.71428571 0.72857143 0.74285714 0.75714286 0.77142857 0.78571429 0.8 0.81428571 0.82857143 0.84285714 0.85714286 0.87142857 0.88571429 0.9 0.91428571 0.92857143 0.94285714 0.95714286 0.97142857 0.98571429 1 1 1 1 1 1
  arc A26 (-14.0526, 10.9042) -> (-14.713, 9.9953) centre (0, 0) ccw
  spline S13 degree 5 poles (-14.713, 9.9953) (-14.7095, 9.9876) (-14.7024, 9.9721) (-14.6918, 9.949) (-14.6775, 9.9183) (-14.6596, 9.8801) (-14.6415, 9.8419) (-14.6232, 9.804) (-14.6048, 9.7661) (-14.5862, 9.7284) (-14.5675, 9.6909) (-14.5486, 9.6535) (-14.5296, 9.6162) (-14.5104, 9.5791) (-14.491, 9.5422) (-14.4716, 9.5054) (-14.4519, 9.4687) (-14.4321, 9.4323) (-14.4121, 9.3959) (-14.392, 9.3597) (-14.3718, 9.3237) (-14.3513, 9.2879) (-14.3307, 9.2522) (-14.31, 9.2166) (-14.2891, 9.1813) (-14.268, 9.1461) (-14.2468, 9.1111) (-14.2254, 9.0762) (-14.2039, 9.0415) (-14.1822, 9.007) (-14.1604, 8.9727) (-14.1383, 8.9386) (-14.1162, 8.9046) (-14.0938, 8.8708) (-14.0713, 8.8372) (-14.0486, 8.8038) (-14.0258, 8.7706) (-14.0028, 8.7376) (-13.9796, 8.7048) (-13.9562, 8.6721) (-13.9327, 8.6397) (-13.909, 8.6075) (-13.8852, 8.5755) (-13.8611, 8.5437) (-13.8369, 8.5122) (-13.8125, 8.4808) (-13.788, 8.4497) (-13.7632, 8.4188) (-13.7383, 8.3881) (-13.7132, 8.3576) (-13.6879, 8.3274) (-13.6624, 8.2975) (-13.6367, 8.2678) (-13.6108, 8.2384) (-13.5847, 8.2093) (-13.5584, 8.1805) (-13.5319, 8.1518) (-13.5052, 8.1235) (-13.4784, 8.0953) (-13.4513, 8.0675) (-13.424, 8.0401) (-13.3963, 8.013) (-13.3684, 7.9864) (-13.3402, 7.9603) (-13.3116, 7.9346) (-13.2829, 7.9091) (-13.2541, 7.8839) (-13.2251, 7.8589) (-13.1959, 7.8342) (-13.1663, 7.8101) (-13.1361, 7.787) (-13.1112, 7.7695) (-13.0921, 7.7571) (-13.0791, 7.7492) (-13.0726, 7.7453) knots -1 -1 -1 -1 -1 -1 -0.98571429 -0.97142857 -0.95714286 -0.94285714 -0.92857143 -0.91428571 -0.9 -0.88571429 -0.87142857 -0.85714286 -0.84285714 -0.82857143 -0.81428571 -0.8 -0.78571429 -0.77142857 -0.75714286 -0.74285714 -0.72857143 -0.71428571 -0.7 -0.68571429 -0.67142857 -0.65714286 -0.64285714 -0.62857143 -0.61428571 -0.6 -0.58571429 -0.57142857 -0.55714286 -0.54285714 -0.52857143 -0.51428571 -0.5 -0.48571429 -0.47142857 -0.45714286 -0.44285714 -0.42857143 -0.41428571 -0.4 -0.38571429 -0.37142857 -0.35714286 -0.34285714 -0.32857143 -0.31428571 -0.3 -0.28571429 -0.27142857 -0.25714286 -0.24285714 -0.22857143 -0.21428571 -0.2 -0.18571429 -0.17142857 -0.15714286 -0.14285714 -0.12857143 -0.11428571 -0.1 -0.08571429 -0.07142857 -0.05714286 -0.04285714 -0.02857143 -0.01428571 0 0 0 0 0 0
  line L13 (-13.0726, 7.7453) -> (-12.5379, 7.4278)
  arc A27 (-12.3925, 6.8895) -> (-12.5379, 7.4278) centre (-12.7421, 7.0839) ccw
  arc A28 (-12.3925, 6.8895) -> (-12.8578, 5.9762) centre (0, 0) ccw
  arc A29 (-13.3788, 5.7774) -> (-12.8578, 5.9762) centre (-13.2206, 6.1448) ccw
  line L14 (-13.3788, 5.7774) -> (-13.95, 6.0234)
  spline S14 degree 5 poles (-13.95, 6.0234) (-13.957, 6.0264) (-13.971, 6.0322) (-13.9923, 6.0404) (-14.021, 6.0502) (-14.0575, 6.0611) (-14.0943, 6.0709) (-14.1315, 6.08) (-14.1687, 6.0888) (-14.2061, 6.0973) (-14.2436, 6.1055) (-14.2812, 6.1135) (-14.3189, 6.121) (-14.3569, 6.1279) (-14.395, 6.1344) (-14.4332, 6.1404) (-14.4717, 6.1459) (-14.5102, 6.1511) (-14.5488, 6.156) (-14.5875, 6.1606) (-14.6264, 6.1649) (-14.6653, 6.1689) (-14.7043, 6.1726) (-14.7434, 6.176) (-14.7826, 6.179) (-14.8219, 6.1817) (-14.8613, 6.1841) (-14.9008, 6.1862) (-14.9403, 6.1881) (-14.9799, 6.1897) (-15.0196, 6.191) (-15.0594, 6.192) (-15.0992, 6.1928) (-15.1392, 6.1933) (-15.1791, 6.1935) (-15.2192, 6.1935) (-15.2593, 6.1932) (-15.2995, 6.1927) (-15.3397, 6.1919) (-15.38, 6.1908) (-15.4204, 6.1895) (-15.4608, 6.188) (-15.5012, 6.1862) (-15.5417, 6.1842) (-15.5823, 6.182) (-15.6229, 6.1795) (-15.6636, 6.1767) (-15.7043, 6.1738) (-15.7451, 6.1706) (-15.7859, 6.1672) (-15.8267, 6.1635) (-15.8676, 6.1596) (-15.9086, 6.1555) (-15.9495, 6.1512) (-15.9906, 6.1466) (-16.0316, 6.1419) (-16.0727, 6.1369) (-16.1138, 6.1317) (-16.155, 6.1262) (-16.1962, 6.1206) (-16.2374, 6.1147) (-16.2787, 6.1087) (-16.32, 6.1024) (-16.3613, 6.0959) (-16.4027, 6.0892) (-16.444, 6.0823) (-16.4854, 6.0751) (-16.5269, 6.0678) (-16.5683, 6.0602) (-16.6098, 6.0525) (-16.6513, 6.0445) (-16.6846, 6.038) (-16.7095, 6.033) (-16.7261, 6.0297) (-16.7344, 6.028) knots 0 0 0 0 0 0 0.01428571 0.02857143 0.04285714 0.05714286 0.07142857 0.08571429 0.1 0.11428571 0.12857143 0.14285714 0.15714286 0.17142857 0.18571429 0.2 0.21428571 0.22857143 0.24285714 0.25714286 0.27142857 0.28571429 0.3 0.31428571 0.32857143 0.34285714 0.35714286 0.37142857 0.38571429 0.4 0.41428571 0.42857143 0.44285714 0.45714286 0.47142857 0.48571429 0.5 0.51428571 0.52857143 0.54285714 0.55714286 0.57142857 0.58571429 0.6 0.61428571 0.62857143 0.64285714 0.65714286 0.67142857 0.68571429 0.7 0.71428571 0.72857143 0.74285714 0.75714286 0.77142857 0.78571429 0.8 0.81428571 0.82857143 0.84285714 0.85714286 0.87142857 0.88571429 0.9 0.91428571 0.92857143 0.94285714 0.95714286 0.97142857 0.98571429 1 1 1 1 1 1
  arc A30 (-16.7344, 6.028) -> (-17.0816, 4.9595) centre (0, 0) ccw
  spline S15 degree 5 poles (-17.0816, 4.9595) (-17.0759, 4.9533) (-17.0644, 4.9408) (-17.0471, 4.9221) (-17.0241, 4.8973) (-16.9952, 4.8664) (-16.9662, 4.8358) (-16.9371, 4.8053) (-16.9079, 4.775) (-16.8786, 4.7449) (-16.8492, 4.715) (-16.8196, 4.6853) (-16.79, 4.6557) (-16.7603, 4.6263) (-16.7305, 4.5972) (-16.7006, 4.5682) (-16.6706, 4.5394) (-16.6405, 4.5108) (-16.6103, 4.4825) (-16.5799, 4.4543) (-16.5495, 4.4263) (-16.519, 4.3985) (-16.4884, 4.3709) (-16.4577, 4.3435) (-16.4269, 4.3163) (-16.396, 4.2894) (-16.365, 4.2626) (-16.3339, 4.2361) (-16.3027, 4.2098) (-16.2714, 4.1836) (-16.24, 4.1577) (-16.2085, 4.1321) (-16.1769, 4.1066) (-16.1452, 4.0814) (-16.1134, 4.0564) (-16.0816, 4.0317) (-16.0496, 4.0071) (-16.0175, 3.9828) (-15.9853, 3.9588) (-15.953, 3.935) (-15.9206, 3.9114) (-15.8882, 3.8881) (-15.8556, 3.865) (-15.8229, 3.8422) (-15.7901, 3.8197) (-15.7572, 3.7974) (-15.7242, 3.7754) (-15.6911, 3.7537) (-15.658, 3.7322) (-15.6247, 3.711) (-15.5913, 3.6901) (-15.5578, 3.6695) (-15.5242, 3.6492) (-15.4904, 3.6293) (-15.4566, 3.6096) (-15.4227, 3.5903) (-15.3886, 3.5713) (-15.3545, 3.5525) (-15.3203, 3.5341) (-15.2859, 3.516) (-15.2515, 3.4983) (-15.2168, 3.4811) (-15.1821, 3.4645) (-15.1471, 3.4484) (-15.112, 3.4327) (-15.0769, 3.4173) (-15.0416, 3.4023) (-15.0063, 3.3874) (-14.9709, 3.373) (-14.9353, 3.3592) (-14.8995, 3.3466) (-14.8704, 3.3376) (-14.8484, 3.3318) (-14.8336, 3.3282) (-14.8262, 3.3266) knots -1 -1 -1 -1 -1 -1 -0.98571429 -0.97142857 -0.95714286 -0.94285714 -0.92857143 -0.91428571 -0.9 -0.88571429 -0.87142857 -0.85714286 -0.84285714 -0.82857143 -0.81428571 -0.8 -0.78571429 -0.77142857 -0.75714286 -0.74285714 -0.72857143 -0.71428571 -0.7 -0.68571429 -0.67142857 -0.65714286 -0.64285714 -0.62857143 -0.61428571 -0.6 -0.58571429 -0.57142857 -0.55714286 -0.54285714 -0.52857143 -0.51428571 -0.5 -0.48571429 -0.47142857 -0.45714286 -0.44285714 -0.42857143 -0.41428571 -0.4 -0.38571429 -0.37142857 -0.35714286 -0.34285714 -0.32857143 -0.31428571 -0.3 -0.28571429 -0.27142857 -0.25714286 -0.24285714 -0.22857143 -0.21428571 -0.2 -0.18571429 -0.17142857 -0.15714286 -0.14285714 -0.12857143 -0.11428571 -0.1 -0.08571429 -0.07142857 -0.05714286 -0.04285714 -0.02857143 -0.01428571 0 0 0 0 0 0
  line L15 (-14.8262, 3.3266) -> (-14.2195, 3.1899)
  arc A31 (-13.9149, 2.7228) -> (-14.2195, 3.1899) centre (-14.3075, 2.7996) ccw
  arc A32 (-13.9149, 2.7228) -> (-14.0753, 1.7104) centre (0, 0) ccw
  arc A33 (-14.5093, 1.3603) -> (-14.0753, 1.7104) centre (-14.4723, 1.7586) ccw
  line L16 (-14.5093, 1.3603) -> (-15.1285, 1.4178)
  spline S16 degree 5 poles (-15.1285, 1.4178) (-15.1361, 1.4185) (-15.1513, 1.4197) (-15.174, 1.4209) (-15.2044, 1.4214) (-15.2424, 1.4204) (-15.2805, 1.4184) (-15.3186, 1.4156) (-15.3568, 1.4124) (-15.395, 1.4089) (-15.4332, 1.4052) (-15.4714, 1.4011) (-15.5096, 1.3966) (-15.5478, 1.3915) (-15.5861, 1.3859) (-15.6243, 1.3797) (-15.6625, 1.3731) (-15.7008, 1.3662) (-15.7391, 1.3589) (-15.7773, 1.3513) (-15.8155, 1.3434) (-15.8538, 1.3352) (-15.892, 1.3266) (-15.9303, 1.3177) (-15.9685, 1.3085) (-16.0067, 1.2989) (-16.0449, 1.2891) (-16.0831, 1.2789) (-16.1213, 1.2684) (-16.1595, 1.2577) (-16.1976, 1.2467) (-16.2358, 1.2354) (-16.2739, 1.2238) (-16.312, 1.2119) (-16.3501, 1.1998) (-16.3882, 1.1874) (-16.4263, 1.1747) (-16.4643, 1.1618) (-16.5023, 1.1486) (-16.5403, 1.1351) (-16.5783, 1.1214) (-16.6163, 1.1075) (-16.6542, 1.0933) (-16.6921, 1.0789) (-16.73, 1.0642) (-16.7678, 1.0493) (-16.8057, 1.0341) (-16.8435, 1.0187) (-16.8813, 1.0031) (-16.919, 0.9872) (-16.9567, 0.9711) (-16.9944, 0.9548) (-17.0321, 0.9382) (-17.0697, 0.9215) (-17.1073, 0.9045) (-17.1449, 0.8872) (-17.1824, 0.8698) (-17.22, 0.8521) (-17.2574, 0.8342) (-17.2949, 0.8161) (-17.3323, 0.7978) (-17.3696, 0.7793) (-17.407, 0.7606) (-17.4443, 0.7416) (-17.4815, 0.7225) (-17.5187, 0.7031) (-17.5559, 0.6835) (-17.593, 0.6637) (-17.6301, 0.6437) (-17.6672, 0.6236) (-17.7042, 0.6032) (-17.7338, 0.5867) (-17.756, 0.5742) (-17.7707, 0.5659) (-17.7781, 0.5617) knots 0 0 0 0 0 0 0.01428571 0.02857143 0.04285714 0.05714286 0.07142857 0.08571429 0.1 0.11428571 0.12857143 0.14285714 0.15714286 0.17142857 0.18571429 0.2 0.21428571 0.22857143 0.24285714 0.25714286 0.27142857 0.28571429 0.3 0.31428571 0.32857143 0.34285714 0.35714286 0.37142857 0.38571429 0.4 0.41428571 0.42857143 0.44285714 0.45714286 0.47142857 0.48571429 0.5 0.51428571 0.52857143 0.54285714 0.55714286 0.57142857 0.58571429 0.6 0.61428571 0.62857143 0.64285714 0.65714286 0.67142857 0.68571429 0.7 0.71428571 0.72857143 0.74285714 0.75714286 0.77142857 0.78571429 0.8 0.81428571 0.82857143 0.84285714 0.85714286 0.87142857 0.88571429 0.9 0.91428571 0.92857143 0.94285714 0.95714286 0.97142857 0.98571429 1 1 1 1 1 1
  arc A34 (-17.7781, 0.5617) -> (-17.7781, -0.5617) centre (0, 0) ccw